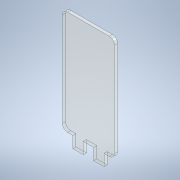
# Autodesk Inventor part: Scheibe
Saved by Autodesk Inventor 2021 (Build 250183000, 183)
## iProperties
Created: 2021-03-05
Part Number: Scheibe
Material: Glas
Document SubType Name: Modeling
Designer: Tilman
Density: 2.18 g/cm^3
Appearance: Klar
Author: Tilman
Autodesk Inventor part; units mm, degrees
ref_plane "YZ Plane" through (0, 0, 0) normal (1, 0, 0) x (0, 1, 0)
ref_plane "XZ Plane" through (0, 0, 0) normal (0, 1, 0) x (-1, 0, 0)
ref_plane "XY Plane" through (0, 0, 0) normal (0, 0, 1) x (1, 0, 0)
sketch "Skizze1" plane through (0, 0, 0) normal (0, 0, 1) x (1, 0, 0)
  line L0 (0, 5) -> (0, 95)
  line L1 (5, 100) -> (45, 100)
  line L2 (50, 95) -> (50, 5)
  arc A0 (5, 100) -> (0, 95) centre (5, 95) ccw
  arc A1 (50, 95) -> (45, 100) centre (45, 95) ccw
  arc A2 (45, 0) -> (50, 5) centre (45, 5) ccw
  arc A3 (0, 5) -> (5, 0) centre (5, 5) ccw
  line L3 (10, 0) -> (10, -11)
  line L4 (10, -11) -> (20, -11)
  line L5 (20, -11) -> (20, 0)
  line L6 (30, 0) -> (30, -11)
  line L7 (30, -11) -> (40, -11)
  line L8 (40, -11) -> (40, 0)
  line L9 (5, 0) -> (10, 0)
  line L10 (20, 0) -> (30, 0)
  line L11 (40, 0) -> (45, 0)
  point P0 (0, 0)
  dimension "d1" = 50
  dimension "d3" = 5
  dimension "d4" = 11
  dimension "d5" = 10
  dimension "d6" = 100
  constraints: 24 end point, 8 point on circle, 7 tangent, 5 equal length, 4 centre point, 4 horizontal, 3 equal radius, 3 horizontal alignment, 3 vertical, 2 collinear, 2 parallel, 1 perpendicular, 1 vertical alignment
  measures "d1" distance between parallel lines of L2 L0
  measures "d3" radius of A0
  measures "d4" distance of L3.start L3.end
  measures "d5" distance of L3.end L4.end
  measures "d6" distance between parallel lines of L10 L1
extrude "Extrusion1" add sketch "Skizze1" along normal blind 3
